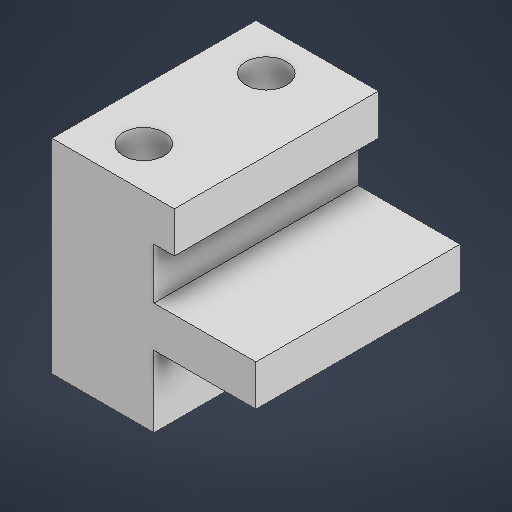
# Autodesk Inventor part: suport1_pcb_temp
Saved by Autodesk Inventor 2026.1 (Build 301233000, 233)
## iProperties
Created: 2025-09-26
Part Number: suport1_pcb_temp
Material: Generic
Document SubType Name: Modeling
Designer: emanuel
Density: 1 g/cm^3
Appearance: Default
Author: emanuel
Autodesk Inventor part; units mm, degrees
ref_plane "YZ Plane" through (0, 0, 0) normal (1, 0, 0) x (0, 1, 0)
ref_plane "XZ Plane" through (0, 0, 0) normal (0, 1, 0) x (-1, 0, 0)
ref_plane "XY Plane" through (0, 0, 0) normal (0, 0, 1) x (1, 0, 0)
sketch "Sketch1" plane through (0, 0, 0) normal (0, 1, 0) x (-1, 0, 0)
  line L0 (0, 0) -> (5, 0)
  line L1 (5, 0) -> (5, -10)
  line L2 (5, -10) -> (0, -10)
  line L3 (0, -10) -> (0, 0)
  dimension "d0" = 5
  dimension "d1" = 10
  constraints: 8 end point, 2 parallel, 1 horizontal, 1 perpendicular
  measures "d0" distance of L1.end L2.end
  measures "d1" distance of L0.end L1.end
extrude "Extrusion1" add sketch "Sketch1" along normal blind 10
sketch "Sketch2" plane through (0, 0, 0) normal (1, 0, 0) x (0, 0, -1)
  line L0 (10, 10) -> (0, 10) projected
  line L1 (10, 0) -> (10, 10) projected
  line L2 (0, 10) -> (10, 10)
  line L3 (10, 10) -> (10, 8)
  line L4 (10, 8) -> (0, 8)
  line L5 (0, 8) -> (0, 10)
  line L6 (0, 8) -> (10, 8)
  line L7 (10, 8) -> (10, 5.5)
  line L8 (10, 5.5) -> (0, 5.5)
  line L9 (0, 5.5) -> (0, 8)
  line L10 (0, 5.5) -> (10, 5.5)
  line L11 (10, 5.5) -> (10, 3.5)
  line L12 (10, 3.5) -> (0, 3.5)
  line L13 (0, 3.5) -> (0, 5.5)
  point P0 (0, 0)
  dimension "d4" = 2
  dimension "d5" = 2.5
  dimension "d6" = 2
  constraints: 24 end point, 6 parallel, 3 horizontal, 3 perpendicular, 3 point on line
  measures "d4" distance of L2.end L3.end
  measures "d5" distance of L6.end L7.end
  measures "d6" distance of L10.end L11.end
extrude "Extrusion2" add sketch "Sketch2" along normal blind 5 contours L1 L4 L5 L0 | L1 L12 L13 L8
sketch "Sketch3" plane through (0, 10, 0) normal (0, 1, 0) x (1, 0, 0)
  line L0 (-5, 10) -> (-5, 0) projected
  line L1 (-5, 0) -> (-2.5, 0)
  line L2 (-2.5, 0) -> (-2.5, 2)
  line L3 (-2.5, 2) -> (-5, 2)
  line L4 (-5, 2) -> (-5, 0)
  line L5 (0, 10) -> (-5, 10) projected
  line L6 (-5, 10) -> (-2.5, 10)
  line L7 (-2.5, 10) -> (-2.5, 8)
  line L8 (-2.5, 8) -> (-5, 8)
  line L9 (-5, 8) -> (-5, 10)
  circle A0 centre (-2.5, 2) radius 1
  circle A1 centre (-2.5, 8) radius 1
  point P0 (0, 0)
  dimension "d9" = 2.5
  dimension "d10" = 2
  dimension "d11" = 2.5
  dimension "d12" = 2
  dimension "d13" = 2
  dimension "d14" = 2
  constraints: 16 end point, 4 parallel, 2 centre point, 2 coincident, 2 horizontal, 2 perpendicular
  measures "d9" distance of L3.end L2.end
  measures "d10" distance of L2.end L1.end
  measures "d11" distance of L7.end L8.end
  measures "d12" distance of L6.end L7.end
  measures "d13" diameter of A0
  measures "d14" diameter of A1
extrude "Extrusion3" cut sketch "Sketch3" against normal blind 20 contours A1 L7 L8 | L8 L7 A1 | A0 L2 L3 | L3 L2 A0
sketch "Sketch4" plane through (5, 0, 0) normal (1, 0, 0) x (0, 0, -1)
  line L0 (0, 10) -> (0, 8) projected
  line L1 (0, 8) -> (10, 8) projected
  line L2 (0, 10) -> (10, 10)
  line L3 (10, 10) -> (10, 8)
  line L4 (10, 8) -> (0, 8)
  line L5 (0, 8) -> (0, 10)
  point P0 (0, 0)
  constraints: 8 end point, 2 parallel, 1 horizontal, 1 perpendicular
extrude "Extrusion4" cut sketch "Sketch4" against normal blind 4
body "Solid1"
